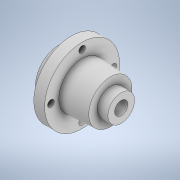
# Autodesk Inventor part: Part2
Saved by Autodesk Inventor 2021 (Build 250183000, 183)
## iProperties
Created: 2022-06-02
Part Number: Part2
Material: Generic
Document SubType Name: Modeling
Designer: Bhargav Malasani
Density: 1 g/cm^3
Appearance: Default
Author: Bhargav Malasani
Autodesk Inventor part; units mm, degrees
ref_plane "YZ Plane" through (0, 0, 0) normal (1, 0, 0) x (0, 1, 0)
ref_plane "XZ Plane" through (0, 0, 0) normal (0, 1, 0) x (-1, 0, 0)
ref_plane "XY Plane" through (0, 0, 0) normal (0, 0, 1) x (1, 0, 0)
sketch "Sketch1" plane through (0, 0, 0) normal (0, 0, 1) x (1, 0, 0)
  line L0 (0, 0) -> (75, 0)
  line L1 (0, 22) -> (54, 22)
  line L2 (0, 28) -> (15, 28)
  line L3 (15, 28) -> (15, 45)
  line L4 (15, 45) -> (28, 45)
  line L5 (28, 45) -> (28, 28)
  line L6 (54, 12) -> (41, 12)
  line L7 (54, 12) -> (54, 22)
  line L8 (41, 8) -> (75, 8)
  line L9 (75, 16) -> (62, 16)
  line L10 (75, 8) -> (75, 16)
  line L11 (62, 16) -> (62, 26)
  line L12 (28, 28) -> (62, 26)
  line L13 (41, 8) -> (41, 12)
  line L14 (0, 22) -> (0, 28)
  dimension "d0" = 75
  dimension "d1" = 54
  dimension "d2" = 22
  dimension "d3" = 15
  dimension "d4" = 17
  dimension "d5" = 13
  dimension "d6" = 28
  dimension "d7" = 13
  dimension "d8" = 12
  dimension "d9" = 8
  dimension "d10" = 13
  dimension "d11" = 16
  dimension "d12" = 26
  dimension "d13" = 15
  dimension "d14" = 54
  dimension "d15" = 62
  constraints: 30 end point, 6 horizontal, 4 vertical, 3 perpendicular, 1 point on line
  measures "d0" distance of L0.start L0.end
  measures "d1" distance of L1.start L1.end
  measures "d2" distance between parallel lines of L0 L1
  measures "d3" distance of L2.start L2.end
  measures "d4" distance of L2.end L3.end
  measures "d5" distance of L3.end L4.end
  measures "d6" distance between parallel lines of L0 L2
  measures "d7" distance of L6.start L6.end
  measures "d8" distance between parallel lines of L0 L6
  measures "d9" distance between parallel lines of L0 L8
  measures "d10" distance of L9.start L9.end
  measures "d11" distance between parallel lines of L0 L9
  measures "d12" distance from line of L0 L11.end
  measures "d13" distance from line of L0.start L3
  measures "d14" distance from line of L0.start L7
  measures "d15" distance from line of L0.start L11
revolve "Revolution1" add sketch "Sketch1" angle 360 about axis through (0, 0, 0) along (1, 0, 0)
sketch "Sketch2" plane through (15, 0, 0) normal (-1, 0, 0) x (0, 0, 1)
  circle A0 centre (0, 37.5) radius 4
  circle A1 centre (-37.5, 0) radius 4
  circle A2 centre (0, -37.5) radius 4
  circle A3 centre (37.5, 0) radius 4
  point P0 (0, 0)
  dimension "d19" = 8
  dimension "d20" = 37.5
  dimension "d23" = 360
  constraints: 4 centre point, 9 other
  measures "d19" diameter of A0
  measures "d20" distance of point (0, 0) A0.centre
extrude "Extrusion1" cut sketch "Sketch2" against normal through all
body "Solid1"
